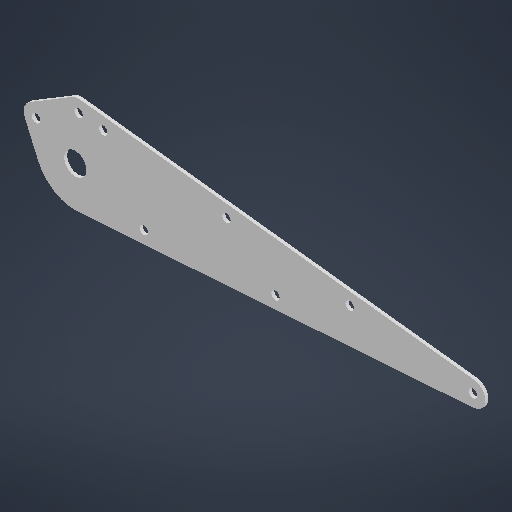
# Autodesk Inventor part: intake
Saved by Autodesk Inventor 2025.1 (Build 291241000, 241)
## iProperties
Created: 2025-01-15
Part Number: intake
Material: Generic
Document SubType Name: Modeling
Designer: Jahan
Density: 1 g/cm^3
Appearance: Default
Author: Jahan
Autodesk Inventor part; units mm, degrees
ref_plane "YZ Plane" through (0, 0, 0) normal (1, 0, 0) x (0, 1, 0)
ref_plane "XZ Plane" through (0, 0, 0) normal (0, 1, 0) x (-1, 0, 0)
ref_plane "XY Plane" through (0, 0, 0) normal (0, 0, 1) x (1, 0, 0)
sketch "Sketch1" plane through (0, 0, 0) normal (0, 0, 1) x (1, 0, 0)
  circle A0 centre (0, 0) radius 5.715
  circle A1 centre (203.2, 0) radius 2.1844
  line L0 (203.6465, -6.3343) -> (1.4511, -20.5864)
  circle A2 centre (1.7066, 23.2882) radius 2.1844
  circle A3 centre (-20.0159, 10.124) radius 2.1844
  line L1 (-23.3069, 15.5547) -> (-1.5845, 28.7188)
  line L2 (-25.8346, 7.5814) -> (-18.9109, -8.2635)
  arc A4 (-23.3069, 15.5547) -> (-25.8346, 7.5814) centre (-20.0159, 10.124) ccw
  line L3 (203.2, 6.35) -> (2.4369, 29.596)
  arc A5 (2.4369, 29.596) -> (-1.5845, 28.7188) centre (1.7066, 23.2882) ccw
  arc A6 (-18.9109, -8.2635) -> (1.4511, -20.5864) centre (0, 0) ccw
  circle A7 centre (14.3223, 21.8274) radius 2.1844
  circle A8 centre (77.2831, 14.5373) radius 2.1844
  circle A9 centre (140.2439, 7.2472) radius 2.1844
  circle A10 centre (35.0777, -11.8662) radius 2.1844
  circle A11 centre (102.3309, -7.1257) radius 2.1844
  arc A12 (203.6465, -6.3343) -> (203.2, 6.35) centre (203.2, 0) ccw
  dimension "d0" = 11.43
  dimension "d3" = 4.3688
  dimension "d30" = 4.3688
  dimension "d36" = 4.3688
  dimension "d45" = 4.3688
  dimension "d47" = 4.3688
  dimension "d51" = 4.3688
  dimension "d52" = 4.3688
  constraints: 13 centre point, 8 end point, 8 point on circle, 2 coincident, 2 tangent
  measures "d0" diameter of A0
  measures "d3" diameter of A1
  measures "d30" diameter of A3
  measures "d36" diameter of A7
  measures "d45" diameter of A8
  measures "d47" diameter of A9
  measures "d51" diameter of A10
  measures "d52" diameter of A11
extrude "Extrusion1" add sketch "Sketch1" along normal blind 1.5875
body "Solid1"
